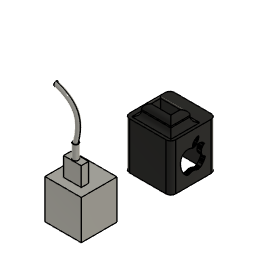
IPad Charger Protector Mini v6 (Autodesk Fusion 360 design; units mm, degrees)
Autodesk Fusion 360 part; units mm, degrees
(part 1 of 2)
sketch "Sketch1" plane through (0, 0, 0) normal (0, 0, 1) x (1, 0, 0)
  line L0 (0, 0) -> (-27, 0)
  line L1 (-27, 0) -> (-27, 26.3)
  line L2 (-27, 26.3) -> (0, 26.3)
  line L3 (0, 26.3) -> (0, 0)
  line L4 (5, -5) -> (-32, -5)
  line L5 (-32, -5) -> (-32, 31.3)
  line L6 (-32, 31.3) -> (5, 31.3)
  line L7 (5, 31.3) -> (5, -5)
  dimension "d1" = 27
  dimension "d2" = 26.3
  dimension "d3" = 37
  dimension "d4" = 36.3
  constraint horizontal L0
  constraint vertical L1
  constraint horizontal L2
  constraint vertical L3
  constraint coincident L0.start L3.end
  constraint horizontal L4
  constraint vertical L5
  constraint horizontal L6
  constraint vertical L7
  measures "d1" distance of L0.start L0.end
  measures "d2" distance of L0.start L2.end
  measures "d3" distance of L4.start L4.end
  measures "d4" distance of L4.start L6.end
extrude "Extrude1" add sketch "Sketch1" along normal blind 28.5 makes body 1
sketch "Sketch2" plane through (0, 0, 28.5) normal (0, 0, 1) x (-1, 0, 0)
  line L0 (27, -26.3) -> (0, -26.3)
  line L1 (0, -26.3) -> (0, 0)
  line L2 (0, 0) -> (27, 0)
  line L3 (27, 0) -> (27, -26.3)
  line L4 (-5, -31.3) -> (32, -31.3)
  line L5 (32, -31.3) -> (32, 5)
  line L6 (32, 5) -> (-5, 5)
  line L7 (-5, 5) -> (-5, -31.3)
  line L8 (6.5, -6.5) -> (19.5, -6.5)
  line L9 (19.5, -6.5) -> (19.5, -12.2)
  line L10 (19.5, -12.2) -> (6.5, -12.2)
  line L11 (6.5, -12.2) -> (6.5, -6.5)
  line L12 (6.5, -6.5) -> (6.5, -4)
  line L13 (6.5, -1.5) -> (1.5, -1.5)
  line L14 (19.5, -17.2) -> (24.5, -17.2)
  line L15 (24.5, -17.2) -> (1.5, -17.2)
  line L16 (1.5, -17.2) -> (1.5, -1.5)
  line L17 (1.5, -1.5) -> (24.5, -1.5)
  line L18 (24.5, -1.5) -> (24.5, -17.2)
  dimension "d9" = 13
  dimension "d10" = 5.7
  dimension "d11" = 5
  dimension "d12" = 5
  dimension "d13" = 5
  dimension "d14" = 5
  constraint horizontal L8
  constraint vertical L9
  constraint horizontal L10
  constraint vertical L11
  constraint perpendicular L8 L12
  constraint horizontal L15
  constraint vertical L16
  constraint horizontal L17
  constraint vertical L18
  measures "d9" distance of L8.start L8.end
  measures "d10" distance of L8.start L10.end
  measures "d11" distance of L8.start L13.start
  measures "d12" distance of L13.start L13.end
  measures "d13" distance of L9.end L14.start
  measures "d14" distance of L14.start L14.end
extrude "Extrude2" add sketch "Sketch2" along normal blind 13 separate body contours L13 L14 L15 L16 L17 L18 makes body 2
sketch "Sketch3" plane through (0, 0, 28.5) normal (0, 0, 1) x (-1, 0, 0)
  line L0 (27, -26.3) -> (0, -26.3)
  line L1 (0, -26.3) -> (0, 0)
  line L2 (0, 0) -> (27, 0)
  line L3 (27, 0) -> (27, -26.3)
  line L4 (-5, -31.3) -> (32, -31.3)
  line L5 (32, -31.3) -> (32, 5)
  line L6 (32, 5) -> (-5, 5)
  line L7 (-5, 5) -> (-5, -31.3)
  line L8 (-5, -31.3) -> (32, -31.3)
  line L9 (32, -31.3) -> (32, 5)
  line L10 (32, 5) -> (-5, 5)
  line L11 (-5, 5) -> (-5, -31.3)
  constraint horizontal L8
  constraint vertical L9
  constraint horizontal L10
  constraint vertical L11
  constraint coincident L5.end L6.start
  constraint coincident L4.start L7.end
extrude "Extrude3" add sketch "Sketch3" along normal blind 5 contours L0 L1 L2 L3 | L4 L5 L6 L7 L8 L9 L10 L11 bodies 2 1
extrude "Extrude4" cut 1 faces at (-10.8333, 10.3, 33.5) along direction (0, 0, -1) blind 5 on bodies 2 bodies 2
sketch "Sketch4" plane through (-32, 0, 0) normal (-1, 0, 0) x (0, -1, 0)
  line L0 (-31.3, 0) -> (5, 0)
  line L1 (5, 0) -> (5, 33.5)
  line L2 (5, 33.5) -> (-31.3, 33.5)
  line L3 (-31.3, 33.5) -> (-31.3, 0)
  spline S0 degree 3 poles (-9.4138, 27.7944) (-9.4601, 27.7871) (-9.5404, 27.7763) (-9.5919, 27.7695) knots 0 0 0 0 1 1 1 1
  spline S1 degree 3 poles (-9.5919, 27.7695) (-9.7044, 27.7554) (-9.8119, 27.739) (-9.8916, 27.7237) knots 0 0 0 0 1 1 1 1
  spline S2 degree 3 poles (-9.8916, 27.7237) (-10.0267, 27.6972) (-10.2931, 27.6248) (-10.4214, 27.5795) knots 0 0 0 0 1 1 1 1
  spline S3 degree 3 poles (-10.4214, 27.5795) (-10.4706, 27.562) (-10.5323, 27.5405) (-10.5589, 27.5309) knots 0 0 0 0 1 1 1 1
  spline S4 degree 3 poles (-10.5589, 27.5309) (-10.5854, 27.5219) (-10.6143, 27.5111) (-10.6239, 27.5066) knots 0 0 0 0 1 1 1 1
  spline S5 degree 3 poles (-10.6239, 27.5066) (-10.6329, 27.5026) (-10.6725, 27.4862) (-10.7115, 27.4698) knots 0 0 0 0 1 1 1 1
  spline S6 degree 3 poles (-10.7115, 27.4698) (-10.7506, 27.4534) (-10.7845, 27.4387) (-10.7879, 27.4359) knots 0 0 0 0 1 1 1 1
  spline S7 degree 3 poles (-10.7879, 27.4359) (-10.7907, 27.4336) (-10.819, 27.4212) (-10.8501, 27.4082) knots 0 0 0 0 1 1 1 1
  spline S8 degree 3 poles (-10.8501, 27.4082) (-10.8812, 27.3946) (-10.9332, 27.3697) (-10.966, 27.3528) knots 0 0 0 0 1 1 1 1
  spline S9 degree 3 poles (-10.966, 27.3528) (-10.9988, 27.3352) (-11.0542, 27.3064) (-11.0887, 27.2883) knots 0 0 0 0 1 1 1 1
  spline S10 degree 3 poles (-11.0887, 27.2883) (-11.1826, 27.2402) (-11.4393, 27.083) (-11.4947, 27.0406) knots 0 0 0 0 1 1 1 1
  spline S11 degree 3 poles (-11.4947, 27.0406) (-11.5072, 27.031) (-11.5366, 27.0101) (-11.5598, 26.9937) knots 0 0 0 0 1 1 1 1
  spline S12 degree 3 poles (-11.5598, 26.9937) (-11.6661, 26.9202) (-11.8182, 26.802) (-11.9358, 26.7013) knots 0 0 0 0 1 1 1 1
  spline S13 degree 3 poles (-11.9358, 26.7013) (-12.0297, 26.6216) (-12.0907, 26.5634) (-12.2299, 26.4237) knots 0 0 0 0 1 1 1 1
  spline S14 degree 3 poles (-12.2299, 26.4237) (-12.4272, 26.2252) (-12.4312, 26.2213) (-12.4962, 26.1466) knots 0 0 0 0 1 1 1 1
  spline S15 degree 3 poles (-12.4962, 26.1466) (-12.6082, 26.0194) (-12.6653, 25.9481) (-12.8196, 25.7451) knots 0 0 0 0 1 1 1 1
  spline S16 degree 3 poles (-12.8196, 25.7451) (-12.8581, 25.6948) (-12.974, 25.5229) (-13.0498, 25.4047) knots 0 0 0 0 1 1 1 1
  spline S17 degree 3 poles (-13.0498, 25.4047) (-13.1363, 25.269) (-13.2822, 24.9896) (-13.3438, 24.8403) knots 0 0 0 0 1 1 1 1
  spline S18 degree 3 poles (-13.3438, 24.8403) (-13.3586, 24.8047) (-13.3766, 24.7629) (-13.3834, 24.747) knots 0 0 0 0 1 1 1 1
  spline S19 degree 3 poles (-13.3834, 24.747) (-13.4027, 24.7029) (-13.4202, 24.6577) (-13.4224, 24.6441) knots 0 0 0 0 1 1 1 1
  spline S20 degree 3 poles (-13.4224, 24.6441) (-13.4241, 24.6373) (-13.4366, 24.6006) (-13.4502, 24.5621) knots 0 0 0 0 1 1 1 1
  spline S21 degree 3 poles (-13.4502, 24.5621) (-13.4711, 24.5033) (-13.4897, 24.4473) (-13.5225, 24.3399) knots 0 0 0 0 1 1 1 1
  spline S22 degree 3 poles (-13.5225, 24.3399) (-13.5254, 24.3308) (-13.5288, 24.3156) (-13.5299, 24.306) knots 0 0 0 0 1 1 1 1
  spline S23 degree 3 poles (-13.5299, 24.306) (-13.531, 24.2969) (-13.5423, 24.2472) (-13.5553, 24.1957) knots 0 0 0 0 1 1 1 1
  spline S24 degree 3 poles (-13.5553, 24.1957) (-13.6011, 24.0085) (-13.6311, 23.8259) (-13.6379, 23.6896) knots 0 0 0 0 1 1 1 1
  spline S25 degree 3 poles (-13.6379, 23.6896) (-13.639, 23.6619) (-13.643, 23.6008) (-13.6458, 23.5539) knots 0 0 0 0 1 1 1 1
  spline S26 degree 3 poles (-13.6458, 23.5539) (-13.6532, 23.447) (-13.6532, 23.2881) (-13.6464, 23.1891) knots 0 0 0 0 1 1 1 1
  spline S27 degree 3 poles (-13.6464, 23.1891) (-13.643, 23.1473) (-13.6396, 23.0862) (-13.6379, 23.0534) knots 0 0 0 0 1 1 1 1
  spline S28 degree 3 poles (-13.6379, 23.0534) (-13.6362, 23.0206) (-13.6294, 22.9409) (-13.6226, 22.8759) knots 0 0 0 0 1 1 1 1
  line L4 (-13.6226, 22.8759) -> (-13.6108, 22.7577)
  line L5 (-13.6108, 22.7577) -> (-13.5056, 22.7616)
  spline S29 degree 3 poles (-13.5056, 22.7616) (-13.259, 22.7707) (-13.013, 22.7978) (-12.784, 22.8419) knots 0 0 0 0 1 1 1 1
  spline S30 degree 3 poles (-12.784, 22.8419) (-12.6427, 22.8691) (-12.3616, 22.9505) (-12.2202, 23.0054) knots 0 0 0 0 1 1 1 1
  spline S31 degree 3 poles (-12.2202, 23.0054) (-12.1592, 23.0285) (-12.1077, 23.0478) (-12.1054, 23.0478) knots 0 0 0 0 1 1 1 1
  spline S32 degree 3 poles (-12.1054, 23.0478) (-12.1032, 23.0478) (-12.0879, 23.054) (-12.0721, 23.0613) knots 0 0 0 0 1 1 1 1
  spline S33 degree 3 poles (-12.0721, 23.0613) (-12.0562, 23.0687) (-12.0189, 23.0857) (-11.9895, 23.0987) knots 0 0 0 0 1 1 1 1
  spline S34 degree 3 poles (-11.9895, 23.0987) (-11.9341, 23.123) (-11.9256, 23.1269) (-11.7973, 23.192) knots 0 0 0 0 1 1 1 1
  spline S35 degree 3 poles (-11.7973, 23.192) (-11.6791, 23.2513) (-11.4076, 23.4102) (-11.3958, 23.4266) knots 0 0 0 0 1 1 1 1
  spline S36 degree 3 poles (-11.3958, 23.4266) (-11.3941, 23.4289) (-11.3647, 23.4498) (-11.3307, 23.473) knots 0 0 0 0 1 1 1 1
  spline S37 degree 3 poles (-11.3307, 23.473) (-11.247, 23.5301) (-11.1475, 23.6031) (-11.0621, 23.6721) knots 0 0 0 0 1 1 1 1
  spline S38 degree 3 poles (-11.0621, 23.6721) (-10.9954, 23.7258) (-10.975, 23.7433) (-10.8676, 23.8411) knots 0 0 0 0 1 1 1 1
  spline S39 degree 3 poles (-10.8676, 23.8411) (-10.7087, 23.9853) (-10.4486, 24.2551) (-10.3293, 24.3993) knots 0 0 0 0 1 1 1 1
  spline S40 degree 3 poles (-10.3293, 24.3993) (-10.2812, 24.4575) (-10.1438, 24.639) (-10.098, 24.7052) knots 0 0 0 0 1 1 1 1
  spline S41 degree 3 poles (-10.098, 24.7052) (-10.0822, 24.7278) (-10.0663, 24.7493) (-10.0624, 24.7533) knots 0 0 0 0 1 1 1 1
  spline S42 degree 3 poles (-10.0624, 24.7533) (-10.0516, 24.7646) (-9.9295, 24.958) (-9.9052, 25.0021) knots 0 0 0 0 1 1 1 1
  spline S43 degree 3 poles (-9.9052, 25.0021) (-9.8938, 25.0236) (-9.8786, 25.049) (-9.8712, 25.0592) knots 0 0 0 0 1 1 1 1
  spline S44 degree 3 poles (-9.8712, 25.0592) (-9.856, 25.0795) (-9.6993, 25.3793) (-9.6993, 25.3877) knots 0 0 0 0 1 1 1 1
  spline S45 degree 3 poles (-9.6993, 25.3877) (-9.6993, 25.3906) (-9.6863, 25.4211) (-9.6705, 25.4545) knots 0 0 0 0 1 1 1 1
  spline S46 degree 3 poles (-9.6705, 25.4545) (-9.6366, 25.5274) (-9.5919, 25.6343) (-9.5885, 25.6512) knots 0 0 0 0 1 1 1 1
  spline S47 degree 3 poles (-9.5885, 25.6512) (-9.5874, 25.658) (-9.584, 25.6682) (-9.5806, 25.6744) knots 0 0 0 0 1 1 1 1
  spline S48 degree 3 poles (-9.5806, 25.6744) (-9.5613, 25.7123) (-9.4924, 25.9142) (-9.4867, 25.9487) knots 0 0 0 0 1 1 1 1
  spline S49 degree 3 poles (-9.4867, 25.9487) (-9.4856, 25.9566) (-9.4805, 25.973) (-9.476, 25.9854) knots 0 0 0 0 1 1 1 1
  spline S50 degree 3 poles (-9.476, 25.9854) (-9.4618, 26.025) (-9.4008, 26.2637) (-9.3883, 26.3264) knots 0 0 0 0 1 1 1 1
  spline S51 degree 3 poles (-9.3883, 26.3264) (-9.3549, 26.5023) (-9.3278, 26.7008) (-9.3108, 26.8846) knots 0 0 0 0 1 1 1 1
  spline S52 degree 3 poles (-9.3108, 26.8846) (-9.2944, 27.0689) (-9.2984, 27.5473) (-9.3182, 27.7712) knots 0 0 0 0 1 1 1 1
  spline S53 degree 3 poles (-9.3182, 27.7712) (-9.3205, 27.7922) (-9.3233, 27.8086) (-9.3255, 27.8086) knots 0 0 0 0 1 1 1 1
  spline S54 degree 3 poles (-9.3255, 27.8086) (-9.3272, 27.808) (-9.3668, 27.8018) (-9.4138, 27.7944) knots 0 0 0 0 1 1 1 1
  spline S55 degree 3 poles (-17.0873, 23.0308) (-17.3757, 23.0144) (-17.6641, 22.981) (-17.9525, 22.9313) knots 0 0 0 0 1 1 1 1
  spline S56 degree 3 poles (-17.9525, 22.9313) (-18.108, 22.9041) (-18.4371, 22.8216) (-18.5972, 22.7701) knots 0 0 0 0 1 1 1 1
  spline S57 degree 3 poles (-18.5972, 22.7701) (-18.751, 22.7204) (-18.8183, 22.6977) (-18.8403, 22.6887) knots 0 0 0 0 1 1 1 1
  spline S58 degree 3 poles (-18.8403, 22.6887) (-18.8494, 22.6842) (-18.9133, 22.6593) (-18.9811, 22.6321) knots 0 0 0 0 1 1 1 1
  spline S59 degree 3 poles (-18.9811, 22.6321) (-19.049, 22.6056) (-19.1282, 22.5722) (-19.1564, 22.5586) knots 0 0 0 0 1 1 1 1
  spline S60 degree 3 poles (-19.1564, 22.5586) (-19.1847, 22.5451) (-19.2407, 22.519) (-19.2814, 22.5004) knots 0 0 0 0 1 1 1 1
  spline S61 degree 3 poles (-19.2814, 22.5004) (-19.3215, 22.4823) (-19.3775, 22.454) (-19.4058, 22.4376) knots 0 0 0 0 1 1 1 1
  spline S62 degree 3 poles (-19.4058, 22.4376) (-19.4335, 22.4218) (-19.4584, 22.4088) (-19.4607, 22.4088) knots 0 0 0 0 1 1 1 1
  spline S63 degree 3 poles (-19.4607, 22.4088) (-19.4759, 22.4088) (-19.8067, 22.2114) (-19.8978, 22.1475) knots 0 0 0 0 1 1 1 1
  spline S64 degree 3 poles (-19.8978, 22.1475) (-20.0708, 22.0271) (-20.2308, 21.9055) (-20.3502, 21.8048) knots 0 0 0 0 1 1 1 1
  spline S65 degree 3 poles (-20.3502, 21.8048) (-20.491, 21.6855) (-20.7941, 21.3853) (-20.919, 21.2405) knots 0 0 0 0 1 1 1 1
  spline S66 degree 3 poles (-20.919, 21.2405) (-21.0236, 21.12) (-21.1068, 21.0154) (-21.204, 20.882) knots 0 0 0 0 1 1 1 1
  spline S67 degree 3 poles (-21.204, 20.882) (-21.2351, 20.8401) (-21.2634, 20.8022) (-21.2674, 20.7983) knots 0 0 0 0 1 1 1 1
  spline S68 degree 3 poles (-21.2674, 20.7983) (-21.2775, 20.7881) (-21.394, 20.6117) (-21.4364, 20.5427) knots 0 0 0 0 1 1 1 1
  spline S69 degree 3 poles (-21.4364, 20.5427) (-21.4545, 20.5133) (-21.4709, 20.4878) (-21.4726, 20.4861) knots 0 0 0 0 1 1 1 1
  spline S70 degree 3 poles (-21.4726, 20.4861) (-21.4879, 20.4743) (-21.6417, 20.1944) (-21.7141, 20.0473) knots 0 0 0 0 1 1 1 1
  spline S71 degree 3 poles (-21.7141, 20.0473) (-21.7967, 19.8805) (-21.8232, 19.8228) (-21.8685, 19.7143) knots 0 0 0 0 1 1 1 1
  spline S72 degree 3 poles (-21.8685, 19.7143) (-21.929, 19.5689) (-21.9431, 19.5339) (-21.9454, 19.522) knots 0 0 0 0 1 1 1 1
  spline S73 degree 3 poles (-21.9454, 19.522) (-21.9465, 19.5158) (-21.9539, 19.4943) (-21.9618, 19.4739) knots 0 0 0 0 1 1 1 1
  spline S74 degree 3 poles (-21.9618, 19.4739) (-21.9833, 19.4213) (-22.0438, 19.2523) (-22.0455, 19.2421) knots 0 0 0 0 1 1 1 1
  spline S75 degree 3 poles (-22.0455, 19.2421) (-22.0466, 19.2376) (-22.0489, 19.2302) (-22.0511, 19.2268) knots 0 0 0 0 1 1 1 1
  spline S76 degree 3 poles (-22.0511, 19.2268) (-22.0539, 19.2229) (-22.0545, 19.2195) (-22.0534, 19.2195) knots 0 0 0 0 1 1 1 1
  spline S77 degree 3 poles (-22.0534, 19.2195) (-22.0517, 19.2195) (-22.0579, 19.1957) (-22.0675, 19.1674) knots 0 0 0 0 1 1 1 1
  spline S78 degree 3 poles (-22.0675, 19.1674) (-22.1088, 19.0368) (-22.1478, 18.9039) (-22.1529, 18.8745) knots 0 0 0 0 1 1 1 1
  spline S79 degree 3 poles (-22.1529, 18.8745) (-22.1546, 18.8666) (-22.1659, 18.8191) (-22.1789, 18.7688) knots 0 0 0 0 1 1 1 1
  spline S80 degree 3 poles (-22.1789, 18.7688) (-22.2168, 18.6184) (-22.257, 18.4346) (-22.262, 18.3916) knots 0 0 0 0 1 1 1 1
  spline S81 degree 3 poles (-22.262, 18.3916) (-22.2632, 18.3792) (-22.2683, 18.3475) (-22.2728, 18.3209) knots 0 0 0 0 1 1 1 1
  spline S82 degree 3 poles (-22.2728, 18.3209) (-22.322, 18.0495) (-22.3621, 17.7464) (-22.3684, 17.605) knots 0 0 0 0 1 1 1 1
  spline S83 degree 3 poles (-22.3684, 17.605) (-22.3701, 17.5711) (-22.3751, 17.4897) (-22.3797, 17.4241) knots 0 0 0 0 1 1 1 1
  spline S84 degree 3 poles (-22.3797, 17.4241) (-22.3961, 17.1956) (-22.4017, 16.9756) (-22.3983, 16.6776) knots 0 0 0 0 1 1 1 1
  spline S85 degree 3 poles (-22.3983, 16.6776) (-22.3949, 16.3955) (-22.3915, 16.3022) (-22.3746, 16.0499) knots 0 0 0 0 1 1 1 1
  spline S86 degree 3 poles (-22.3746, 16.0499) (-22.3706, 15.9815) (-22.3667, 15.9114) (-22.3667, 15.8944) knots 0 0 0 0 1 1 1 1
  spline S87 degree 3 poles (-22.3667, 15.8944) (-22.3661, 15.8062) (-22.3129, 15.355) (-22.2756, 15.1169) knots 0 0 0 0 1 1 1 1
  spline S88 degree 3 poles (-22.2756, 15.1169) (-22.27, 15.0796) (-22.2632, 15.0315) (-22.2615, 15.0106) knots 0 0 0 0 1 1 1 1
  spline S89 degree 3 poles (-22.2615, 15.0106) (-22.2587, 14.9772) (-22.2411, 14.8749) (-22.2106, 14.7126) knots 0 0 0 0 1 1 1 1
  spline S90 degree 3 poles (-22.2106, 14.7126) (-22.2055, 14.686) (-22.1914, 14.6165) (-22.1789, 14.5571) knots 0 0 0 0 1 1 1 1
  spline S91 degree 3 poles (-22.1789, 14.5571) (-22.167, 14.4983) (-22.1557, 14.4389) (-22.1546, 14.4265) knots 0 0 0 0 1 1 1 1
  spline S92 degree 3 poles (-22.1546, 14.4265) (-22.1518, 14.3987) (-22.1331, 14.3156) (-22.0907, 14.1443) knots 0 0 0 0 1 1 1 1
  spline S93 degree 3 poles (-22.0907, 14.1443) (-22.0737, 14.0759) (-22.0562, 14.0023) (-22.0523, 13.9803) knots 0 0 0 0 1 1 1 1
  spline S94 degree 3 poles (-22.0523, 13.9803) (-22.0415, 13.926) (-22.0008, 13.7739) (-21.9539, 13.6144) knots 0 0 0 0 1 1 1 1
  spline S95 degree 3 poles (-21.9539, 13.6144) (-21.9476, 13.5929) (-21.9442, 13.576) (-21.9459, 13.576) knots 0 0 0 0 1 1 1 1
  spline S96 degree 3 poles (-21.9459, 13.576) (-21.9476, 13.576) (-21.9459, 13.5726) (-21.9425, 13.5686) knots 0 0 0 0 1 1 1 1
  spline S97 degree 3 poles (-21.9425, 13.5686) (-21.9392, 13.5641) (-21.9375, 13.5596) (-21.9392, 13.5579) knots 0 0 0 0 1 1 1 1
  spline S98 degree 3 poles (-21.9392, 13.5579) (-21.942, 13.555) (-21.929, 13.5109) (-21.8702, 13.3272) knots 0 0 0 0 1 1 1 1
  spline S99 degree 3 poles (-21.8702, 13.3272) (-21.8526, 13.2729) (-21.8379, 13.2231) (-21.8368, 13.2169) knots 0 0 0 0 1 1 1 1
  spline S100 degree 3 poles (-21.8368, 13.2169) (-21.8362, 13.2107) (-21.8125, 13.1389) (-21.7842, 13.0569) knots 0 0 0 0 1 1 1 1
  spline S101 degree 3 poles (-21.7842, 13.0569) (-21.7559, 12.9749) (-21.7316, 12.9025) (-21.7305, 12.8957) knots 0 0 0 0 1 1 1 1
  spline S102 degree 3 poles (-21.7305, 12.8957) (-21.7277, 12.8833) (-21.6836, 12.7605) (-21.6457, 12.6605) knots 0 0 0 0 1 1 1 1
  spline S103 degree 3 poles (-21.6457, 12.6605) (-21.6344, 12.6316) (-21.6253, 12.605) (-21.6253, 12.6016) knots 0 0 0 0 1 1 1 1
  spline S104 degree 3 poles (-21.6253, 12.6016) (-21.6253, 12.5988) (-21.5999, 12.5321) (-21.5693, 12.4541) knots 0 0 0 0 1 1 1 1
  spline S105 degree 3 poles (-21.5693, 12.4541) (-21.5382, 12.376) (-21.5043, 12.2895) (-21.493, 12.2612) knots 0 0 0 0 1 1 1 1
  spline S106 degree 3 poles (-21.493, 12.2612) (-21.4822, 12.2335) (-21.4591, 12.1775) (-21.4415, 12.1368) knots 0 0 0 0 1 1 1 1
  spline S107 degree 3 poles (-21.4415, 12.1368) (-21.424, 12.0967) (-21.4087, 12.0588) (-21.4076, 12.0537) knots 0 0 0 0 1 1 1 1
  spline S108 degree 3 poles (-21.4076, 12.0537) (-21.4065, 12.0486) (-21.3889, 12.0079) (-21.3692, 11.9632) knots 0 0 0 0 1 1 1 1
  spline S109 degree 3 poles (-21.3692, 11.9632) (-21.3494, 11.9185) (-21.3143, 11.8405) (-21.2917, 11.7891) knots 0 0 0 0 1 1 1 1
  spline S110 degree 3 poles (-21.2917, 11.7891) (-21.2691, 11.7376) (-21.2397, 11.6731) (-21.2255, 11.6449) knots 0 0 0 0 1 1 1 1
  spline S111 degree 3 poles (-21.2255, 11.6449) (-21.2114, 11.6171) (-21.1989, 11.5894) (-21.1978, 11.5838) knots 0 0 0 0 1 1 1 1
  spline S112 degree 3 poles (-21.1978, 11.5838) (-21.1933, 11.5578) (-20.8619, 10.8979) (-20.8014, 10.7938) knots 0 0 0 0 1 1 1 1
  spline S113 degree 3 poles (-20.8014, 10.7938) (-20.7918, 10.7768) (-20.7737, 10.7435) (-20.7618, 10.7203) knots 0 0 0 0 1 1 1 1
  spline S114 degree 3 poles (-20.7618, 10.7203) (-20.7211, 10.6434) (-20.6566, 10.5252) (-20.647, 10.5111) knots 0 0 0 0 1 1 1 1
  spline S115 degree 3 poles (-20.647, 10.5111) (-20.6419, 10.5031) (-20.6176, 10.4613) (-20.5933, 10.4178) knots 0 0 0 0 1 1 1 1
  spline S116 degree 3 poles (-20.5933, 10.4178) (-20.569, 10.3742) (-20.5413, 10.3256) (-20.5317, 10.3098) knots 0 0 0 0 1 1 1 1
  spline S117 degree 3 poles (-20.5317, 10.3098) (-20.5221, 10.2934) (-20.5, 10.2566) (-20.4825, 10.2278) knots 0 0 0 0 1 1 1 1
  spline S118 degree 3 poles (-20.4825, 10.2278) (-20.4649, 10.1984) (-20.4401, 10.1554) (-20.4265, 10.1322) knots 0 0 0 0 1 1 1 1
  spline S119 degree 3 poles (-20.4265, 10.1322) (-20.4129, 10.109) (-20.3897, 10.0711) (-20.3745, 10.0485) knots 0 0 0 0 1 1 1 1
  spline S120 degree 3 poles (-20.3745, 10.0485) (-20.3598, 10.0259) (-20.3473, 10.0067) (-20.3473, 10.005) knots 0 0 0 0 1 1 1 1
  spline S121 degree 3 poles (-20.3473, 10.005) (-20.3473, 10.0038) (-20.323, 9.9637) (-20.2936, 9.9167) knots 0 0 0 0 1 1 1 1
  spline S122 degree 3 poles (-20.2936, 9.9167) (-20.2642, 9.8698) (-20.2399, 9.8302) (-20.2399, 9.8291) knots 0 0 0 0 1 1 1 1
  spline S123 degree 3 poles (-20.2399, 9.8291) (-20.2399, 9.8274) (-20.1975, 9.7629) (-20.1641, 9.7137) knots 0 0 0 0 1 1 1 1
  spline S124 degree 3 poles (-20.1641, 9.7137) (-20.1568, 9.703) (-20.1172, 9.6419) (-20.0753, 9.578) knots 0 0 0 0 1 1 1 1
  spline S125 degree 3 poles (-20.0753, 9.578) (-20.0341, 9.5141) (-19.9826, 9.4378) (-19.9611, 9.4084) knots 0 0 0 0 1 1 1 1
  spline S126 degree 3 poles (-19.9611, 9.4084) (-19.9402, 9.379) (-19.8876, 9.3049) (-19.8446, 9.2444) knots 0 0 0 0 1 1 1 1
  spline S127 degree 3 poles (-19.8446, 9.2444) (-19.766, 9.1324) (-19.6942, 9.0357) (-19.6376, 8.9645) knots 0 0 0 0 1 1 1 1
  spline S128 degree 3 poles (-19.6376, 8.9645) (-19.6201, 8.943) (-19.58, 8.8921) (-19.5483, 8.8514) knots 0 0 0 0 1 1 1 1
  spline S129 degree 3 poles (-19.5483, 8.8514) (-19.4437, 8.7174) (-19.2831, 8.5262) (-19.2135, 8.4527) knots 0 0 0 0 1 1 1 1
  spline S130 degree 3 poles (-19.2135, 8.4527) (-18.9568, 8.1824) (-18.8064, 8.036) (-18.6577, 7.911) knots 0 0 0 0 1 1 1 1
  spline S131 degree 3 poles (-18.6577, 7.911) (-18.4501, 7.7368) (-18.2341, 7.5836) (-18.0498, 7.4795) knots 0 0 0 0 1 1 1 1
  spline S132 degree 3 poles (-18.0498, 7.4795) (-18.0255, 7.4659) (-17.9887, 7.445) (-17.9678, 7.4332) knots 0 0 0 0 1 1 1 1
  spline S133 degree 3 poles (-17.9678, 7.4332) (-17.9469, 7.4207) (-17.8994, 7.397) (-17.862, 7.38) knots 0 0 0 0 1 1 1 1
  spline S134 degree 3 poles (-17.862, 7.38) (-17.8247, 7.363) (-17.7914, 7.3466) (-17.7885, 7.3438) knots 0 0 0 0 1 1 1 1
  spline S135 degree 3 poles (-17.7885, 7.3438) (-17.7789, 7.3365) (-17.6907, 7.2991) (-17.6528, 7.2867) knots 0 0 0 0 1 1 1 1
  spline S136 degree 3 poles (-17.6528, 7.2867) (-17.6342, 7.2805) (-17.611, 7.272) (-17.6019, 7.2675) knots 0 0 0 0 1 1 1 1
  spline S137 degree 3 poles (-17.6019, 7.2675) (-17.5544, 7.246) (-17.3763, 7.1889) (-17.3294, 7.1804) knots 0 0 0 0 1 1 1 1
  spline S138 degree 3 poles (-17.3294, 7.1804) (-17.3147, 7.1781) (-17.2672, 7.1679) (-17.2247, 7.1589) knots 0 0 0 0 1 1 1 1
  spline S139 degree 3 poles (-17.2247, 7.1589) (-16.946, 7.0967) (-16.6491, 7.0905) (-16.3041, 7.1385) knots 0 0 0 0 1 1 1 1
  spline S140 degree 3 poles (-16.3041, 7.1385) (-16.2227, 7.1498) (-16.0717, 7.1776) (-15.9931, 7.1951) knots 0 0 0 0 1 1 1 1
  spline S141 degree 3 poles (-15.9931, 7.1951) (-15.897, 7.2171) (-15.625, 7.3008) (-15.5701, 7.3251) knots 0 0 0 0 1 1 1 1
  spline S142 degree 3 poles (-15.5701, 7.3251) (-15.5526, 7.3331) (-15.4667, 7.3687) (-15.3796, 7.4049) knots 0 0 0 0 1 1 1 1
  spline S143 degree 3 poles (-15.3796, 7.4049) (-15.2925, 7.4405) (-15.2184, 7.4716) (-15.2156, 7.4739) knots 0 0 0 0 1 1 1 1
  spline S144 degree 3 poles (-15.2156, 7.4739) (-15.2122, 7.4761) (-15.1947, 7.484) (-15.176, 7.4908) knots 0 0 0 0 1 1 1 1
  spline S145 degree 3 poles (-15.176, 7.4908) (-15.1573, 7.4982) (-15.1104, 7.5168) (-15.0714, 7.5321) knots 0 0 0 0 1 1 1 1
  spline S146 degree 3 poles (-15.0714, 7.5321) (-15.0324, 7.5479) (-14.947, 7.579) (-14.882, 7.6017) knots 0 0 0 0 1 1 1 1
  spline S147 degree 3 poles (-14.882, 7.6017) (-14.8164, 7.6243) (-14.7451, 7.6497) (-14.7236, 7.6576) knots 0 0 0 0 1 1 1 1
  spline S148 degree 3 poles (-14.7236, 7.6576) (-14.6558, 7.6837) (-14.5721, 7.7131) (-14.5455, 7.7204) knots 0 0 0 0 1 1 1 1
  spline S149 degree 3 poles (-14.5455, 7.7204) (-14.5314, 7.7244) (-14.4686, 7.7442) (-14.4058, 7.7645) knots 0 0 0 0 1 1 1 1
  spline S150 degree 3 poles (-14.4058, 7.7645) (-14.2831, 7.8047) (-13.9512, 7.8889) (-13.8273, 7.9121) knots 0 0 0 0 1 1 1 1
  spline S151 degree 3 poles (-13.8273, 7.9121) (-13.7504, 7.9263) (-13.5338, 7.9557) (-13.4287, 7.9664) knots 0 0 0 0 1 1 1 1
  spline S152 degree 3 poles (-13.4287, 7.9664) (-13.1725, 7.9924) (-12.8078, 7.9811) (-12.4985, 7.9381) knots 0 0 0 0 1 1 1 1
  spline S153 degree 3 poles (-12.4985, 7.9381) (-12.4566, 7.9325) (-12.408, 7.9263) (-12.391, 7.924) knots 0 0 0 0 1 1 1 1
  spline S154 degree 3 poles (-12.391, 7.924) (-12.339, 7.9183) (-12.1614, 7.8771) (-12.0715, 7.8505) knots 0 0 0 0 1 1 1 1
  spline S155 degree 3 poles (-12.0715, 7.8505) (-12.0246, 7.8363) (-11.9737, 7.8211) (-11.9573, 7.8165) knots 0 0 0 0 1 1 1 1
  spline S156 degree 3 poles (-11.9573, 7.8165) (-11.9409, 7.812) (-11.8849, 7.7917) (-11.8329, 7.7707) knots 0 0 0 0 1 1 1 1
  spline S157 degree 3 poles (-11.8329, 7.7707) (-11.7809, 7.7504) (-11.7198, 7.7278) (-11.6983, 7.7204) knots 0 0 0 0 1 1 1 1
  spline S158 degree 3 poles (-11.6983, 7.7204) (-11.6762, 7.7131) (-11.6191, 7.6916) (-11.5711, 7.6723) knots 0 0 0 0 1 1 1 1
  spline S159 degree 3 poles (-11.5711, 7.6723) (-11.523, 7.6537) (-11.4653, 7.6316) (-11.4438, 7.6237) knots 0 0 0 0 1 1 1 1
  spline S160 degree 3 poles (-11.4438, 7.6237) (-11.3528, 7.5904) (-11.324, 7.5796) (-11.2996, 7.5689) knots 0 0 0 0 1 1 1 1
  spline S161 degree 3 poles (-11.2996, 7.5689) (-11.2629, 7.5525) (-10.9745, 7.4439) (-10.8981, 7.4173) knots 0 0 0 0 1 1 1 1
  spline S162 degree 3 poles (-10.8981, 7.4173) (-10.7375, 7.3625) (-10.6137, 7.3212) (-10.5617, 7.3059) knots 0 0 0 0 1 1 1 1
  spline S163 degree 3 poles (-10.5617, 7.3059) (-10.228, 7.2064) (-9.9713, 7.1504) (-9.6937, 7.117) knots 0 0 0 0 1 1 1 1
  spline S164 degree 3 poles (-9.6937, 7.117) (-9.6026, 7.1057) (-9.3459, 7.108) (-9.2588, 7.1199) knots 0 0 0 0 1 1 1 1
  spline S165 degree 3 poles (-9.2588, 7.1199) (-9.0722, 7.1465) (-8.8698, 7.2007) (-8.7227, 7.2629) knots 0 0 0 0 1 1 1 1
  spline S166 degree 3 poles (-8.7227, 7.2629) (-8.6905, 7.2765) (-8.6611, 7.2878) (-8.6571, 7.2878) knots 0 0 0 0 1 1 1 1
  spline S167 degree 3 poles (-8.6571, 7.2878) (-8.6492, 7.2878) (-8.3925, 7.4156) (-8.345, 7.4433) knots 0 0 0 0 1 1 1 1
  spline S168 degree 3 poles (-8.345, 7.4433) (-8.3292, 7.4524) (-8.3026, 7.4693) (-8.2851, 7.4812) knots 0 0 0 0 1 1 1 1
  spline S169 degree 3 poles (-8.2851, 7.4812) (-8.2675, 7.4931) (-8.2511, 7.5027) (-8.2494, 7.5027) knots 0 0 0 0 1 1 1 1
  spline S170 degree 3 poles (-8.2494, 7.5027) (-8.2426, 7.5027) (-8.0781, 7.6096) (-8.0266, 7.6469) knots 0 0 0 0 1 1 1 1
  spline S171 degree 3 poles (-8.0266, 7.6469) (-7.9322, 7.7153) (-7.9198, 7.7249) (-7.8564, 7.773) knots 0 0 0 0 1 1 1 1
  spline S172 degree 3 poles (-7.8564, 7.773) (-7.4634, 8.0733) (-7.0574, 8.4736) (-6.6452, 8.9673) knots 0 0 0 0 1 1 1 1
  spline S173 degree 3 poles (-6.6452, 8.9673) (-6.4365, 9.2178) (-6.3194, 9.3671) (-6.1832, 9.5565) knots 0 0 0 0 1 1 1 1
  spline S174 degree 3 poles (-6.1832, 9.5565) (-6.1549, 9.5956) (-6.1266, 9.634) (-6.1198, 9.6414) knots 0 0 0 0 1 1 1 1
  spline S175 degree 3 poles (-6.1198, 9.6414) (-6.1063, 9.6578) (-6.0752, 9.7019) (-5.9813, 9.841) knots 0 0 0 0 1 1 1 1
  spline S176 degree 3 poles (-5.9813, 9.841) (-5.9434, 9.897) (-5.9021, 9.9569) (-5.8891, 9.9739) knots 0 0 0 0 1 1 1 1
  spline S177 degree 3 poles (-5.8891, 9.9739) (-5.8761, 9.9908) (-5.8654, 10.0067) (-5.8654, 10.0089) knots 0 0 0 0 1 1 1 1
  spline S178 degree 3 poles (-5.8654, 10.0089) (-5.8654, 10.0112) (-5.8416, 10.0491) (-5.8128, 10.0937) knots 0 0 0 0 1 1 1 1
  spline S179 degree 3 poles (-5.8128, 10.0937) (-5.7834, 10.1384) (-5.7585, 10.1774) (-5.7574, 10.1814) knots 0 0 0 0 1 1 1 1
  spline S180 degree 3 poles (-5.7574, 10.1814) (-5.7562, 10.1848) (-5.7342, 10.2204) (-5.7082, 10.2606) knots 0 0 0 0 1 1 1 1
  spline S181 degree 3 poles (-5.7082, 10.2606) (-5.6601, 10.3341) (-5.5498, 10.5184) (-5.5442, 10.5337) knots 0 0 0 0 1 1 1 1
  spline S182 degree 3 poles (-5.5442, 10.5337) (-5.5425, 10.5382) (-5.5357, 10.5501) (-5.5289, 10.5591) knots 0 0 0 0 1 1 1 1
  spline S183 degree 3 poles (-5.5289, 10.5591) (-5.5131, 10.5812) (-5.4712, 10.6547) (-5.435, 10.7242) knots 0 0 0 0 1 1 1 1
  spline S184 degree 3 poles (-5.435, 10.7242) (-5.4186, 10.7548) (-5.4005, 10.787) (-5.3943, 10.7955) knots 0 0 0 0 1 1 1 1
  spline S185 degree 3 poles (-5.3943, 10.7955) (-5.3615, 10.843) (-5.0143, 11.5323) (-5.0087, 11.5623) knots 0 0 0 0 1 1 1 1
  spline S186 degree 3 poles (-5.0087, 11.5623) (-5.0075, 11.5674) (-4.9974, 11.5906) (-4.986, 11.6138) knots 0 0 0 0 1 1 1 1
  spline S187 degree 3 poles (-4.986, 11.6138) (-4.9561, 11.6748) (-4.9159, 11.7647) (-4.904, 11.7975) knots 0 0 0 0 1 1 1 1
  spline S188 degree 3 poles (-4.904, 11.7975) (-4.8944, 11.823) (-4.8741, 11.8699) (-4.8187, 11.9938) knots 0 0 0 0 1 1 1 1
  spline S189 degree 3 poles (-4.8187, 11.9938) (-4.8096, 12.0141) (-4.8006, 12.0362) (-4.7994, 12.0418) knots 0 0 0 0 1 1 1 1
  spline S190 degree 3 poles (-4.7994, 12.0418) (-4.7983, 12.0475) (-4.7842, 12.0837) (-4.7683, 12.1227) knots 0 0 0 0 1 1 1 1
  spline S191 degree 3 poles (-4.7683, 12.1227) (-4.7191, 12.2414) (-4.6903, 12.3149) (-4.6926, 12.3149) knots 0 0 0 0 1 1 1 1
  spline S192 degree 3 poles (-4.6926, 12.3149) (-4.6948, 12.3149) (-4.6762, 12.3658) (-4.6665, 12.3856) knots 0 0 0 0 1 1 1 1
  spline S193 degree 3 poles (-4.6665, 12.3856) (-4.6632, 12.3919) (-4.6501, 12.4252) (-4.6377, 12.4591) knots 0 0 0 0 1 1 1 1
  spline S194 degree 3 poles (-4.6377, 12.4591) (-4.6247, 12.4936) (-4.6072, 12.54) (-4.5987, 12.5626) knots 0 0 0 0 1 1 1 1
  spline S195 degree 3 poles (-4.5987, 12.5626) (-4.5896, 12.5847) (-4.584, 12.6033) (-4.5851, 12.6033) knots 0 0 0 0 1 1 1 1
  spline S196 degree 3 poles (-4.5851, 12.6033) (-4.5862, 12.6033) (-4.5795, 12.6254) (-4.5698, 12.652) knots 0 0 0 0 1 1 1 1
  spline S197 degree 3 poles (-4.5698, 12.652) (-4.5602, 12.6786) (-4.5534, 12.7017) (-4.5546, 12.7023) knots 0 0 0 0 1 1 1 1
  spline S198 degree 3 poles (-4.5546, 12.7023) (-4.5557, 12.7034) (-4.5732, 12.7119) (-4.5936, 12.721) knots 0 0 0 0 1 1 1 1
  spline S199 degree 3 poles (-4.5936, 12.721) (-4.614, 12.73) (-4.6643, 12.7572) (-4.705, 12.7809) knots 0 0 0 0 1 1 1 1
  spline S200 degree 3 poles (-4.705, 12.7809) (-4.7463, 12.8047) (-4.7813, 12.8239) (-4.7836, 12.8239) knots 0 0 0 0 1 1 1 1
  spline S201 degree 3 poles (-4.7836, 12.8239) (-4.7887, 12.8239) (-4.8854, 12.8793) (-4.9278, 12.907) knots 0 0 0 0 1 1 1 1
  spline S202 degree 3 poles (-4.9278, 12.907) (-4.9487, 12.9206) (-4.9668, 12.9313) (-4.9691, 12.9313) knots 0 0 0 0 1 1 1 1
  spline S203 degree 3 poles (-4.9691, 12.9313) (-4.9764, 12.9313) (-5.1602, 13.0472) (-5.2767, 13.1247) knots 0 0 0 0 1 1 1 1
  spline S204 degree 3 poles (-5.2767, 13.1247) (-5.4401, 13.2344) (-5.5035, 13.2791) (-5.5826, 13.3413) knots 0 0 0 0 1 1 1 1
  spline S205 degree 3 poles (-5.5826, 13.3413) (-5.6024, 13.3571) (-5.6482, 13.3922) (-5.6838, 13.4205) knots 0 0 0 0 1 1 1 1
  spline S206 degree 3 poles (-5.6838, 13.4205) (-5.9038, 13.5907) (-6.1555, 13.8231) (-6.3325, 14.0199) knots 0 0 0 0 1 1 1 1
  spline S207 degree 3 poles (-6.3325, 14.0199) (-6.51, 14.2178) (-6.7057, 14.4802) (-6.8301, 14.6866) knots 0 0 0 0 1 1 1 1
  spline S208 degree 3 poles (-6.8301, 14.6866) (-6.8482, 14.7171) (-6.8708, 14.7539) (-6.8798, 14.7686) knots 0 0 0 0 1 1 1 1
  spline S209 degree 3 poles (-6.8798, 14.7686) (-6.8889, 14.7827) (-6.9087, 14.8189) (-6.9239, 14.8483) knots 0 0 0 0 1 1 1 1
  spline S210 degree 3 poles (-6.9239, 14.8483) (-6.9398, 14.8777) (-6.9686, 14.9326) (-6.9878, 14.9699) knots 0 0 0 0 1 1 1 1
  spline S211 degree 3 poles (-6.9878, 14.9699) (-7.0076, 15.0072) (-7.0331, 15.0592) (-7.0444, 15.0852) knots 0 0 0 0 1 1 1 1
  spline S212 degree 3 poles (-7.0444, 15.0852) (-7.0557, 15.1118) (-7.071, 15.1463) (-7.0789, 15.1616) knots 0 0 0 0 1 1 1 1
  spline S213 degree 3 poles (-7.0789, 15.1616) (-7.0981, 15.1995) (-7.1349, 15.2882) (-7.14, 15.3086) knots 0 0 0 0 1 1 1 1
  spline S214 degree 3 poles (-7.14, 15.3086) (-7.1422, 15.3171) (-7.149, 15.3352) (-7.1547, 15.3482) knots 0 0 0 0 1 1 1 1
  spline S215 degree 3 poles (-7.1547, 15.3482) (-7.1778, 15.3968) (-7.2429, 15.5795) (-7.2474, 15.6077) knots 0 0 0 0 1 1 1 1
  spline S216 degree 3 poles (-7.2474, 15.6077) (-7.2491, 15.6174) (-7.2553, 15.6411) (-7.2615, 15.6598) knots 0 0 0 0 1 1 1 1
  spline S217 degree 3 poles (-7.2615, 15.6598) (-7.2949, 15.7616) (-7.3503, 15.9793) (-7.3548, 16.0256) knots 0 0 0 0 1 1 1 1
  spline S218 degree 3 poles (-7.3548, 16.0256) (-7.356, 16.042) (-7.3605, 16.0686) (-7.3639, 16.0839) knots 0 0 0 0 1 1 1 1
  spline S219 degree 3 poles (-7.3639, 16.0839) (-7.3746, 16.1302) (-7.3961, 16.2592) (-7.4086, 16.3468) knots 0 0 0 0 1 1 1 1
  spline S220 degree 3 poles (-7.4086, 16.3468) (-7.4775, 16.8439) (-7.4645, 17.3686) (-7.3724, 17.8165) knots 0 0 0 0 1 1 1 1
  spline S221 degree 3 poles (-7.3724, 17.8165) (-7.3616, 17.868) (-7.3543, 17.9115) (-7.356, 17.9138) knots 0 0 0 0 1 1 1 1
  spline S222 degree 3 poles (-7.356, 17.9138) (-7.3571, 17.916) (-7.356, 17.9194) (-7.3526, 17.9217) knots 0 0 0 0 1 1 1 1
  spline S223 degree 3 poles (-7.3526, 17.9217) (-7.3492, 17.924) (-7.3481, 17.9273) (-7.3498, 17.9302) knots 0 0 0 0 1 1 1 1
  spline S224 degree 3 poles (-7.3498, 17.9302) (-7.3537, 17.9364) (-7.3141, 18.0891) (-7.2779, 18.2073) knots 0 0 0 0 1 1 1 1
  spline S225 degree 3 poles (-7.2779, 18.2073) (-7.2627, 18.2587) (-7.2485, 18.3062) (-7.2474, 18.313) knots 0 0 0 0 1 1 1 1
  spline S226 degree 3 poles (-7.2474, 18.313) (-7.244, 18.3311) (-7.2033, 18.4425) (-7.1711, 18.5239) knots 0 0 0 0 1 1 1 1
  spline S227 degree 3 poles (-7.1711, 18.5239) (-7.1552, 18.5629) (-7.1417, 18.5991) (-7.1405, 18.6042) knots 0 0 0 0 1 1 1 1
  spline S228 degree 3 poles (-7.1405, 18.6042) (-7.1343, 18.6336) (-6.9912, 18.9328) (-6.9234, 19.0572) knots 0 0 0 0 1 1 1 1
  spline S229 degree 3 poles (-6.9234, 19.0572) (-6.8714, 19.1527) (-6.7961, 19.2743) (-6.7051, 19.4095) knots 0 0 0 0 1 1 1 1
  spline S230 degree 3 poles (-6.7051, 19.4095) (-6.6197, 19.5361) (-6.5066, 19.6871) (-6.4308, 19.7765) knots 0 0 0 0 1 1 1 1
  spline S231 degree 3 poles (-6.4308, 19.7765) (-6.199, 20.049) (-6.0514, 20.2028) (-5.8286, 20.4047) knots 0 0 0 0 1 1 1 1
  spline S232 degree 3 poles (-5.8286, 20.4047) (-5.7726, 20.4556) (-5.6375, 20.5721) (-5.5883, 20.6117) knots 0 0 0 0 1 1 1 1
  spline S233 degree 3 poles (-5.5883, 20.6117) (-5.5741, 20.623) (-5.5527, 20.6411) (-5.5408, 20.653) knots 0 0 0 0 1 1 1 1
  spline S234 degree 3 poles (-5.5408, 20.653) (-5.4995, 20.6908) (-5.2812, 20.856) (-5.1608, 20.9402) knots 0 0 0 0 1 1 1 1
  spline S235 degree 3 poles (-5.1608, 20.9402) (-5.102, 20.9815) (-5.098, 20.9855) (-5.1093, 21.0024) knots 0 0 0 0 1 1 1 1
  spline S236 degree 3 poles (-5.1093, 21.0024) (-5.1223, 21.0228) (-5.2275, 21.1495) (-5.3021, 21.2354) knots 0 0 0 0 1 1 1 1
  spline S237 degree 3 poles (-5.3021, 21.2354) (-5.5521, 21.5221) (-5.8552, 21.8037) (-6.134, 22.0067) knots 0 0 0 0 1 1 1 1
  spline S238 degree 3 poles (-6.134, 22.0067) (-6.1651, 22.0293) (-6.1933, 22.0514) (-6.1967, 22.0559) knots 0 0 0 0 1 1 1 1
  spline S239 degree 3 poles (-6.1967, 22.0559) (-6.2018, 22.0621) (-6.3409, 22.156) (-6.4823, 22.2487) knots 0 0 0 0 1 1 1 1
  spline S240 degree 3 poles (-6.4823, 22.2487) (-6.5151, 22.2697) (-6.7158, 22.3862) (-6.765, 22.4122) knots 0 0 0 0 1 1 1 1
  spline S241 degree 3 poles (-6.765, 22.4122) (-6.8199, 22.4416) (-7.067, 22.5626) (-7.1094, 22.5807) knots 0 0 0 0 1 1 1 1
  spline S242 degree 3 poles (-7.1094, 22.5807) (-7.136, 22.5926) (-7.1677, 22.6067) (-7.1801, 22.6118) knots 0 0 0 0 1 1 1 1
  spline S243 degree 3 poles (-7.1801, 22.6118) (-7.2135, 22.6271) (-7.43, 22.7113) (-7.4628, 22.7221) knots 0 0 0 0 1 1 1 1
  spline S244 degree 3 poles (-7.4628, 22.7221) (-7.4781, 22.7271) (-7.5454, 22.7492) (-7.6121, 22.7713) knots 0 0 0 0 1 1 1 1
  spline S245 degree 3 poles (-7.6121, 22.7713) (-7.8106, 22.8363) (-8.1522, 22.9194) (-8.3309, 22.946) knots 0 0 0 0 1 1 1 1
  spline S246 degree 3 poles (-8.3309, 22.946) (-8.354, 22.9494) (-8.4112, 22.9584) (-8.4581, 22.9658) knots 0 0 0 0 1 1 1 1
  spline S247 degree 3 poles (-8.4581, 22.9658) (-8.6159, 22.9907) (-8.7719, 23.0082) (-8.9925, 23.0257) knots 0 0 0 0 1 1 1 1
  spline S248 degree 3 poles (-8.9925, 23.0257) (-9.1146, 23.0353) (-9.567, 23.0387) (-9.714, 23.0314) knots 0 0 0 0 1 1 1 1
  spline S249 degree 3 poles (-9.714, 23.0314) (-10.0188, 23.0161) (-10.34, 22.9788) (-10.6295, 22.9256) knots 0 0 0 0 1 1 1 1
  spline S250 degree 3 poles (-10.6295, 22.9256) (-10.7918, 22.8962) (-11.0876, 22.8221) (-11.2403, 22.7735) knots 0 0 0 0 1 1 1 1
  spline S251 degree 3 poles (-11.2403, 22.7735) (-11.3053, 22.7526) (-11.3664, 22.7334) (-11.376, 22.7311) knots 0 0 0 0 1 1 1 1
  spline S252 degree 3 poles (-11.376, 22.7311) (-11.4026, 22.7238) (-11.4653, 22.7011) (-11.5513, 22.6678) knots 0 0 0 0 1 1 1 1
  spline S253 degree 3 poles (-11.5513, 22.6678) (-11.5948, 22.6502) (-11.6468, 22.6304) (-11.6672, 22.6237) knots 0 0 0 0 1 1 1 1
  spline S254 degree 3 poles (-11.6672, 22.6237) (-11.6876, 22.6169) (-11.7509, 22.5926) (-11.8086, 22.5699) knots 0 0 0 0 1 1 1 1
  spline S255 degree 3 poles (-11.8086, 22.5699) (-11.8662, 22.5473) (-11.9234, 22.5258) (-11.9358, 22.5219) knots 0 0 0 0 1 1 1 1
  spline S256 degree 3 poles (-11.9358, 22.5219) (-11.9482, 22.5179) (-11.994, 22.5004) (-12.0376, 22.484) knots 0 0 0 0 1 1 1 1
  spline S257 degree 3 poles (-12.0376, 22.484) (-12.0811, 22.467) (-12.1422, 22.4433) (-12.1733, 22.4314) knots 0 0 0 0 1 1 1 1
  spline S258 degree 3 poles (-12.1733, 22.4314) (-12.2044, 22.4195) (-12.2525, 22.4014) (-12.2807, 22.3918) knots 0 0 0 0 1 1 1 1
  spline S259 degree 3 poles (-12.2807, 22.3918) (-12.3085, 22.3816) (-12.3418, 22.3692) (-12.3543, 22.3635) knots 0 0 0 0 1 1 1 1
  spline S260 degree 3 poles (-12.3543, 22.3635) (-12.4577, 22.3177) (-12.8157, 22.2148) (-12.9265, 22.1996) knots 0 0 0 0 1 1 1 1
  spline S261 degree 3 poles (-12.9265, 22.1996) (-13.0651, 22.1809) (-13.0962, 22.1769) (-13.1652, 22.1707) knots 0 0 0 0 1 1 1 1
  spline S262 degree 3 poles (-13.1652, 22.1707) (-13.2579, 22.1628) (-13.4422, 22.1673) (-13.5135, 22.1792) knots 0 0 0 0 1 1 1 1
  spline S263 degree 3 poles (-13.5135, 22.1792) (-13.5412, 22.1843) (-13.583, 22.1911) (-13.6057, 22.1939) knots 0 0 0 0 1 1 1 1
  spline S264 degree 3 poles (-13.6057, 22.1939) (-13.6566, 22.2018) (-13.7883, 22.2374) (-13.8895, 22.2714) knots 0 0 0 0 1 1 1 1
  spline S265 degree 3 poles (-13.8895, 22.2714) (-13.9314, 22.2855) (-13.9772, 22.3002) (-13.9913, 22.3042) knots 0 0 0 0 1 1 1 1
  spline S266 degree 3 poles (-13.9913, 22.3042) (-14.0055, 22.3081) (-14.0564, 22.3268) (-14.1044, 22.3466) knots 0 0 0 0 1 1 1 1
  spline S267 degree 3 poles (-14.1044, 22.3466) (-14.1525, 22.3658) (-14.2266, 22.3952) (-14.2684, 22.4116) knots 0 0 0 0 1 1 1 1
  spline S268 degree 3 poles (-14.2684, 22.4116) (-14.3103, 22.4286) (-14.377, 22.4557) (-14.416, 22.4727) knots 0 0 0 0 1 1 1 1
  spline S269 degree 3 poles (-14.416, 22.4727) (-14.4556, 22.4902) (-14.4997, 22.5083) (-14.515, 22.5134) knots 0 0 0 0 1 1 1 1
  spline S270 degree 3 poles (-14.515, 22.5134) (-14.5302, 22.5185) (-14.55, 22.5264) (-14.5596, 22.5304) knots 0 0 0 0 1 1 1 1
  spline S271 degree 3 poles (-14.5596, 22.5304) (-14.5964, 22.5479) (-14.7428, 22.6084) (-14.7802, 22.622) knots 0 0 0 0 1 1 1 1
  spline S272 degree 3 poles (-14.7802, 22.622) (-14.8017, 22.6299) (-14.8424, 22.6463) (-14.8706, 22.6587) knots 0 0 0 0 1 1 1 1
  spline S273 degree 3 poles (-14.8706, 22.6587) (-14.9227, 22.6813) (-15.0228, 22.7209) (-15.0742, 22.7396) knots 0 0 0 0 1 1 1 1
  spline S274 degree 3 poles (-15.0742, 22.7396) (-15.1687, 22.7735) (-15.3451, 22.8329) (-15.3739, 22.8402) knots 0 0 0 0 1 1 1 1
  spline S275 degree 3 poles (-15.3739, 22.8402) (-15.3926, 22.8453) (-15.4395, 22.8583) (-15.4785, 22.8696) knots 0 0 0 0 1 1 1 1
  spline S276 degree 3 poles (-15.4785, 22.8696) (-15.5871, 22.9007) (-15.7285, 22.9347) (-15.7794, 22.9409) knots 0 0 0 0 1 1 1 1
  spline S277 degree 3 poles (-15.7794, 22.9409) (-15.8048, 22.9437) (-15.8274, 22.9477) (-15.8297, 22.9494) knots 0 0 0 0 1 1 1 1
  spline S278 degree 3 poles (-15.8297, 22.9494) (-15.8376, 22.9539) (-16.0661, 22.9907) (-16.1599, 23.002) knots 0 0 0 0 1 1 1 1
  spline S279 degree 3 poles (-16.1599, 23.002) (-16.3714, 23.028) (-16.4461, 23.0319) (-16.7283, 23.0336) knots 0 0 0 0 1 1 1 1
  spline S280 degree 3 poles (-16.7283, 23.0336) (-16.8792, 23.0348) (-17.0404, 23.0331) (-17.0873, 23.0308) knots 0 0 0 0 1 1 1 1
sketch "Sketch5" plane through (5, 0, 0) normal (1, 0, 0) x (0, 1, 0)
  line L0 (-5, 0) -> (31.3, 0)
  line L1 (31.3, 0) -> (31.3, 33.5)
  line L2 (31.3, 33.5) -> (-5, 33.5)
  line L3 (-5, 33.5) -> (-5, 0)
extrude "Extrude9" cut 1 faces at (-10.8333, 12.2, 32.8333) along direction (0, 1, 0) blind 0.5 on bodies 2 bodies 2
extrude "Extrude10" cut 1 faces at (-19.5, 8.5667, 32.8333) along direction (-1, 0, 0) blind 0.5 on bodies 2 bodies 2
extrude "Extrude11" cut 1 faces at (-11, 6.5, 37.1667) along direction (0, -1, 0) blind 0.5 on bodies 2 bodies 2
extrude "Extrude12" cut 1 faces at (-6.5, 8.2333, 32.8333) along direction (1, 0, 0) blind 0.5 on bodies 2 bodies 2
sketch "Sketch6" plane through (0, -5, 0) normal (0, -1, 0) x (1, 0, 0)
  line L0 (-32, 0) -> (5, 0)
  line L1 (5, 0) -> (5, 33.5)
  line L2 (5, 33.5) -> (-32, 33.5)
  line L3 (-32, 33.5) -> (-32, 0)
extrude "Extrude13" cut 1 faces at (-7.3333, -5, 11.1667) along direction (0, 1, 0) blind 2 on bodies 2 bodies 2
extrude "Extrude14" cut 1 faces at (-19.6667, 31.3, 11.1667) along direction (0, -1, 0) blind 2 on bodies 2 bodies 2
extrude "Extrude15" cut 1 faces at (5, 18.5333, 22.3333) along direction (-1, 0, 0) blind 2 on bodies 2 bodies 2
extrude "Extrude16" cut sketch "Sketch4" against normal blind 2 bodies 2
extrude "Extrude17" cut sketch "Sketch4" against normal blind 2 contours S0 S1 S2 S3 S4 S5 S6 S7 S8 S9 S10 S11 S12 S13 S14 S15 S16 S17 S18 S19 S20 S21 S22 S23 S24 S25 S26 S27 S28 L4 L5 S29 S30 S31 S32 S33 S34 S35 S36 S37 S38 S39 S40 S41 S42 S43 S44 S45 S46 S47 S48 S49 S50 S51 S52 S53 S54 | S55 S56 S57 S58 S59 S60 S61 S62 S63 S64 S65 S66 S67 S68 S69 S70 S71 S72 S73 S74 S75 S76 S77 S78 S79 S80 S81 S82 S83 S84 S85 S86 S87 S88 S89 S90 S91 S92 S93 S94 S95 S96 S97 S98 S99 S100 S101 S102 S103 S104 S105 S106 S107 S108 S109 S110 S111 S112 S113 S114 S115 S116 S117 S118 S119 S120 S121 S122 S123 S124 S125 S126 S127 S128 S129 S130 S131 S132 S133 S134 S135 S136 S137 S138 S139 S140 S141 S142 S143 S144 S145 S146 S147 S148 S149 S150 S151 S152 S153 S154 S155 S156 S157 S158 S159 S160 S161 S162 S163 S164 S165 S166 S167 S168 S169 S170 S171 S172 S173 S174 S175 S176 S177 S178 S179 S180 S181 S182 S183 S184 S185 S186 S187 S188 S189 S190 S191 S192 S193 S194 S195 S196 S197 S198 S199 S200 S201 S202 S203 S204 S205 S206 S207 S208 S209 S210 S211 S212 S213 S214 S215 S216 S217 S218 S219 S220 S221 S222 S223 S224 S225 S226 S227 S228 S229 S230 S231 S232 S233 S234 S235 S236 S237 S238 S239 S240 S241 S242 S243 S244 S245 S246 S247 S248 S249 S250 S251 S252 S253 S254 S255 S256 S257 S258 S259 S260 S261 S262 S263 S264 S265 S266 S267 S268 S269 S270 S271 S272 S273 S274 S275 S276 S277 S278 S279 S280 bodies 2
extrude "Extrude18" cut sketch "Sketch4" against normal blind 5 contours S0 S1 S2 S3 S4 S5 S6 S7 S8 S9 S10 S11 S12 S13 S14 S15 S16 S17 S18 S19 S20 S21 S22 S23 S24 S25 S26 S27 S28 L4 L5 S29 S30 S31 S32 S33 S34 S35 S36 S37 S38 S39 S40 S41 S42 S43 S44 S45 S46 S47 S48 S49 S50 S51 S52 S53 S54 | S55 S56 S57 S58 S59 S60 S61 S62 S63 S64 S65 S66 S67 S68 S69 S70 S71 S72 S73 S74 S75 S76 S77 S78 S79 S80 S81 S82 S83 S84 S85 S86 S87 S88 S89 S90 S91 S92 S93 S94 S95 S96 S97 S98 S99 S100 S101 S102 S103 S104 S105 S106 S107 S108 S109 S110 S111 S112 S113 S114 S115 S116 S117 S118 S119 S120 S121 S122 S123 S124 S125 S126 S127 S128 S129 S130 S131 S132 S133 S134 S135 S136 S137 S138 S139 S140 S141 S142 S143 S144 S145 S146 S147 S148 S149 S150 S151 S152 S153 S154 S155 S156 S157 S158 S159 S160 S161 S162 S163 S164 S165 S166 S167 S168 S169 S170 S171 S172 S173 S174 S175 S176 S177 S178 S179 S180 S181 S182 S183 S184 S185 S186 S187 S188 S189 S190 S191 S192 S193 S194 S195 S196 S197 S198 S199 S200 S201 S202 S203 S204 S205 S206 S207 S208 S209 S210 S211 S212 S213 S214 S215 S216 S217 S218 S219 S220 S221 S222 S223 S224 S225 S226 S227 S228 S229 S230 S231 S232 S233 S234 S235 S236 S237 S238 S239 S240 S241 S242 S243 S244 S245 S246 S247 S248 S249 S250 S251 S252 S253 S254 S255 S256 S257 S258 S259 S260 S261 S262 S263 S264 S265 S266 S267 S268 S269 S270 S271 S272 S273 S274 S275 S276 S277 S278 S279 S280 bodies 2
extrude "Extrude19" cut 1 faces at (-24.5, 6.7333, 36.1667) along direction (1, 0, 0) blind 1 on bodies 2 bodies 2
extrude "Extrude20" cut 1 faces at (-16.1667, 17.2, 38.8333) along direction (0, -1, 0) blind 1 on bodies 2 bodies 2
extrude "Extrude21" cut 1 faces at (-16.1667, 1.5, 36.1667) along direction (0, 1, 0) blind 1 on bodies 2 bodies 2
extrude "Extrude22" cut 1 faces at (-1.5, 11.6333, 36.1667) along direction (-1, 0, 0) blind 1 on bodies 2 bodies 2